Autodesk Inventor part; units mm, degrees
(part 2 of 2)
  line L844 (-48.1002, -67.2416) -> (-49.6002, -66.3756)
  line L845 (-49.6002, -66.3756) -> (-49.6002, -64.6435)
  line L846 (-42.6002, -64.6435) -> (-42.6002, -66.3756)
  line L847 (-44.1002, -63.7775) -> (-42.6002, -64.6435)
  line L848 (-42.6002, -66.3756) -> (-44.1002, -67.2416)
  line L849 (-45.6002, -64.6435) -> (-44.1002, -63.7775)
  line L850 (-44.1002, -67.2416) -> (-45.6002, -66.3756)
  line L851 (-45.6002, -66.3756) -> (-45.6002, -64.6435)
  line L852 (-38.6002, -64.6435) -> (-38.6002, -66.3756)
  line L853 (-40.1002, -63.7775) -> (-38.6002, -64.6435)
  line L854 (-38.6002, -66.3756) -> (-40.1002, -67.2416)
  line L855 (-41.6002, -64.6435) -> (-40.1002, -63.7775)
  line L856 (-40.1002, -67.2416) -> (-41.6002, -66.3756)
  line L857 (-41.6002, -66.3756) -> (-41.6002, -64.6435)
  point P0 (0, 0)
  point P1 (-72.1002, -29.5096)
  point P2 (-70.6002, -29.5096)
  point P3 (-68.1002, -29.5096)
  point P4 (-66.6002, -29.5096)
  point P5 (-64.1002, -29.5096)
  point P6 (-62.6002, -29.5096)
  point P7 (-60.1002, -29.5096)
  point P8 (-58.6002, -29.5096)
  point P9 (-56.1002, -29.5096)
  point P10 (-54.6002, -29.5096)
  point P11 (-52.1002, -29.5096)
  point P12 (-50.6002, -29.5096)
  point P13 (-48.1002, -29.5096)
  point P14 (-46.6002, -29.5096)
  point P15 (-44.1002, -29.5096)
  point P16 (-42.6002, -29.5096)
  point P17 (-40.1002, -29.5096)
  point P18 (-38.6002, -29.5096)
  point P19 (-36.1002, -29.5096)
  point P20 (-34.6002, -29.5096)
  point P21 (-32.1002, -29.5096)
  point P22 (-30.6002, -29.5096)
  point P23 (-28.1002, -29.5096)
  point P24 (-26.6002, -29.5096)
  point P25 (-24.1002, -29.5096)
  point P26 (-22.6002, -29.5096)
  point P27 (-20.1002, -29.5096)
  point P28 (-18.6002, -29.5096)
  point P29 (-16.1002, -29.5096)
  point P30 (-14.6002, -29.5096)
  point P31 (-12.1002, -29.5096)
  point P32 (-10.6002, -29.5096)
  point P33 (-8.1002, -29.5096)
  point P34 (-6.6002, -29.5096)
  point P35 (-72.1002, -33.5096)
  point P36 (-70.6002, -33.5096)
  point P37 (-68.1002, -33.5096)
  point P38 (-66.6002, -33.5096)
  point P39 (-64.1002, -33.5096)
  point P40 (-62.6002, -33.5096)
  point P41 (-60.1002, -33.5096)
  point P42 (-58.6002, -33.5096)
  point P43 (-56.1002, -33.5096)
  point P44 (-54.6002, -33.5096)
  point P45 (-52.1002, -33.5096)
  point P46 (-50.6002, -33.5096)
  point P47 (-48.1002, -33.5096)
  point P48 (-46.6002, -33.5096)
  point P49 (-44.1002, -33.5096)
  point P50 (-42.6002, -33.5096)
  point P51 (-40.1002, -33.5096)
  point P52 (-38.6002, -33.5096)
  point P53 (-36.1002, -33.5096)
  point P54 (-34.6002, -33.5096)
  point P55 (-32.1002, -33.5096)
  point P56 (-30.6002, -33.5096)
  point P57 (-28.1002, -33.5096)
  point P58 (-26.6002, -33.5096)
  point P59 (-24.1002, -33.5096)
  point P60 (-22.6002, -33.5096)
  point P61 (-20.1002, -33.5096)
  point P62 (-18.6002, -33.5096)
  point P63 (-16.1002, -33.5096)
  point P64 (-14.6002, -33.5096)
  point P65 (-12.1002, -33.5096)
  point P66 (-10.6002, -33.5096)
  point P67 (-8.1002, -33.5096)
  point P68 (-6.6002, -33.5096)
  point P69 (-72.1002, -37.5096)
  point P70 (-70.6002, -37.5096)
  point P71 (-68.1002, -37.5096)
  point P72 (-66.6002, -37.5096)
  point P73 (-64.1002, -37.5096)
  point P74 (-62.6002, -37.5096)
  point P75 (-60.1002, -37.5096)
  point P76 (-58.6002, -37.5096)
  point P77 (-56.1002, -37.5096)
  point P78 (-54.6002, -37.5096)
  point P79 (-52.1002, -37.5096)
  point P80 (-50.6002, -37.5096)
  point P81 (-48.1002, -37.5096)
  point P82 (-46.6002, -37.5096)
  point P83 (-44.1002, -37.5096)
  point P84 (-42.6002, -37.5096)
  point P85 (-40.1002, -37.5096)
  point P86 (-38.6002, -37.5096)
  point P87 (-36.1002, -37.5096)
  point P88 (-34.6002, -37.5096)
  point P89 (-32.1002, -37.5096)
  point P90 (-30.6002, -37.5096)
  point P91 (-28.1002, -37.5096)
  point P92 (-26.6002, -37.5096)
  point P93 (-24.1002, -37.5096)
  point P94 (-22.6002, -37.5096)
  point P95 (-20.1002, -37.5096)
  point P96 (-18.6002, -37.5096)
  point P97 (-16.1002, -37.5096)
  point P98 (-14.6002, -37.5096)
  point P99 (-12.1002, -37.5096)
  point P100 (-10.6002, -37.5096)
  point P101 (-8.1002, -37.5096)
  point P102 (-6.6002, -37.5096)
  point P103 (-72.1002, -41.5096)
  point P104 (-70.6002, -41.5096)
  point P105 (-68.1002, -41.5096)
  point P106 (-66.6002, -41.5096)
  point P107 (-64.1002, -41.5096)
  point P108 (-62.6002, -41.5096)
  point P109 (-60.1002, -41.5096)
  point P110 (-58.6002, -41.5096)
  point P111 (-56.1002, -41.5096)
  point P112 (-54.6002, -41.5096)
  point P113 (-52.1002, -41.5096)
  point P114 (-50.6002, -41.5096)
  point P115 (-48.1002, -41.5096)
  point P116 (-46.6002, -41.5096)
  point P117 (-44.1002, -41.5096)
  point P118 (-42.6002, -41.5096)
  point P119 (-40.1002, -41.5096)
  point P120 (-38.6002, -41.5096)
  point P121 (-36.1002, -41.5096)
  point P122 (-34.6002, -41.5096)
  point P123 (-32.1002, -41.5096)
  point P124 (-30.6002, -41.5096)
  point P125 (-28.1002, -41.5096)
  point P126 (-26.6002, -41.5096)
  point P127 (-24.1002, -41.5096)
  point P128 (-22.6002, -41.5096)
  point P129 (-20.1002, -41.5096)
  point P130 (-18.6002, -41.5096)
  point P131 (-16.1002, -41.5096)
  point P132 (-14.6002, -41.5096)
  point P133 (-12.1002, -41.5096)
  point P134 (-10.6002, -41.5096)
  point P135 (-8.1002, -41.5096)
  point P136 (-6.6002, -41.5096)
  point P137 (-72.1002, -45.5096)
  point P138 (-70.6002, -45.5096)
  point P139 (-68.1002, -45.5096)
  point P140 (-66.6002, -45.5096)
  point P141 (-64.1002, -45.5096)
  point P142 (-62.6002, -45.5096)
  point P143 (-60.1002, -45.5096)
  point P144 (-58.6002, -45.5096)
  point P145 (-56.1002, -45.5096)
  point P146 (-54.6002, -45.5096)
  point P147 (-52.1002, -45.5096)
  point P148 (-50.6002, -45.5096)
  point P149 (-48.1002, -45.5096)
  point P150 (-46.6002, -45.5096)
  point P151 (-44.1002, -45.5096)
  point P152 (-42.6002, -45.5096)
  point P153 (-40.1002, -45.5096)
  point P154 (-38.6002, -45.5096)
  point P155 (-36.1002, -45.5096)
  point P156 (-34.6002, -45.5096)
  point P157 (-32.1002, -45.5096)
  point P158 (-30.6002, -45.5096)
  point P159 (-28.1002, -45.5096)
  point P160 (-26.6002, -45.5096)
  point P161 (-24.1002, -45.5096)
  point P162 (-22.6002, -45.5096)
  point P163 (-20.1002, -45.5096)
  point P164 (-18.6002, -45.5096)
  point P165 (-16.1002, -45.5096)
  point P166 (-14.6002, -45.5096)
  point P167 (-12.1002, -45.5096)
  point P168 (-10.6002, -45.5096)
  point P169 (-8.1002, -45.5096)
  point P170 (-6.6002, -45.5096)
  point P171 (-66.6002, -45.5096)
  point P172 (-68.1002, -45.5096)
  point P173 (-62.6002, -45.5096)
  point P174 (-64.1002, -45.5096)
  point P175 (-58.6002, -45.5096)
  point P176 (-60.1002, -45.5096)
  point P177 (-54.6002, -45.5096)
  point P178 (-56.1002, -45.5096)
  point P179 (-50.6002, -45.5096)
  point P180 (-52.1002, -45.5096)
  point P181 (-46.6002, -45.5096)
  point P182 (-48.1002, -45.5096)
  point P183 (-42.6002, -45.5096)
  point P184 (-44.1002, -45.5096)
  point P185 (-38.6002, -45.5096)
  point P186 (-40.1002, -45.5096)
  point P187 (-70.6002, -49.5096)
  point P188 (-72.1002, -49.5096)
  point P189 (-66.6002, -49.5096)
  point P190 (-68.1002, -49.5096)
  point P191 (-62.6002, -49.5096)
  point P192 (-64.1002, -49.5096)
  point P193 (-58.6002, -49.5096)
  point P194 (-60.1002, -49.5096)
  point P195 (-54.6002, -49.5096)
  point P196 (-56.1002, -49.5096)
  point P197 (-50.6002, -49.5096)
  point P198 (-52.1002, -49.5096)
  point P199 (-46.6002, -49.5096)
  dimension "d5" = 31
  dimension "d6" = 24
  dimension "d7" = 7
  dimension "d8" = 4
  dimension "d9" = 7.5
  dimension "d10" = 5
  dimension "d11" = 4
  dimension "d12" = 9
  dimension "d13" = 4
  dimension "d14" = 4
  dimension "d15" = 3
  dimension "d16" = 3
  dimension "d31" = 5
  dimension "d32" = 3
  dimension "d33" = 5
  dimension "d36" = 4
  dimension "d39" = 4
  dimension "d44" = 4
  dimension "d47" = 4
  constraints: 1672 end point, 5 horizontal, 3 perpendicular, 2 centre point, 2 parallel, 2 vertical, 1 coincident, 1 midpoint, 1931 other
  measures "d5" distance of L1.end L2.end
  measures "d6" distance of L0.end L1.end
  measures "d7" distance between parallel lines of L15 L2
  measures "d8" distance between parallel lines of L17 L1
  measures "d9" diameter of A4
  measures "d10" diameter of A5
  measures "d11" distance from line of A4.centre L3
  measures "d12" distance from line of A4.centre L15
  measures "d13" distance between parallel lines of L0 L26
  measures "d14" distance between parallel lines of L2 L27
  measures "d15" distance between parallel lines of L3 L28
  measures "d16" distance between parallel lines of L1 L29
  measures "d31" distance from line of L11 point (-72.1, -29.51)
  measures "d32" distance between parallel lines of L35 L32
  measures "d33" distance from line of point (-72.1, -29.51) L7
  measures "d36" distance of L30.end L36.start
  measures "d39" distance of L30.end L132.start
  measures "d44" distance of L441.start L540.start
  measures "d47" distance of L441.start L588.start
extrude "Wyciągnięcie proste2" add sketch "Szkic2" along normal blind 3.5 contours L0 L1 L2 L3
chamfer "Faza1" distance 5 angle 45 2 edges at (31.6002, -53.0096, -1.75) (6.6002, -53.0096, -1.75)
fillet "Zaokrąglenie2" radius 1.5 10 edges at (34.6002, -49.0096, -1.75) (3.6002, -49.0096, -1.75) (6.6002, -58.0096, -1.75) (6.6002, -69.0096, -1.75) (3.6002, -73.0096, -1.75) (34.6002, -73.0096, -1.75) (31.6002, -69.0096, -1.75) (31.6002, -58.0096, -1.75) (26.6002, -53.0096, -1.75) (11.6002, -53.0096, -1.75)
sketch "Szkic3" plane through (0, 0, 0) normal (0, 0, -1) x (-1, 0, 0)
  arc A0 (-11.1608, -53.4489) -> (-12.2215, -53.0096) centre (-12.2215, -54.5096) ccw projected
  line L0 (-12.2215, -53.0096) -> (-25.9788, -53.0096) projected
  arc A1 (-25.9788, -53.0096) -> (-27.0395, -53.4489) centre (-25.9788, -54.5096) ccw projected
  line L1 (-27.0395, -53.4489) -> (-31.1608, -57.5702) projected
  arc A2 (-31.1608, -57.5702) -> (-31.6002, -58.6309) centre (-30.1002, -58.6309) ccw projected
  line L2 (-31.6002, -58.6309) -> (-31.6002, -67.5096) projected
  arc A3 (-31.6002, -67.5096) -> (-30.1002, -69.0096) centre (-30.1002, -67.5096) ccw projected
  line L3 (-30.1002, -69.0096) -> (-8.1002, -69.0096) projected
  arc A4 (-8.1002, -69.0096) -> (-6.6002, -67.5096) centre (-8.1002, -67.5096) ccw projected
  line L4 (-6.6002, -67.5096) -> (-6.6002, -58.6309) projected
  arc A5 (-6.6002, -58.6309) -> (-7.0395, -57.5702) centre (-8.1002, -58.6309) ccw projected
  line L5 (-7.0395, -57.5702) -> (-11.1608, -53.4489) projected
  point P0 (0, 0)
extrude "Wyciągnięcie proste3" cut sketch "Szkic3" against normal blind 17
extrude "Wyciągnięcie proste4" add sketch "Szkic2" along normal blind 1 contours A4
extrude "Wyciągnięcie proste5" add sketch "Szkic2" along normal blind 5 contours A5
fillet "Zaokrąglenie3" radius 2.5 1 edges at (41.1002, -71.0096, -5)
extrude "Wyciągnięcie proste6" cut sketch "Szkic2" against normal blind 2 contours L30 L31 L32 L33 L34 L35 | L36 L38 L40 L41 L39 L37 | L42 L44 L46 L47 L45 L43 | L48 L50 L52 L53 L51 L49 | L54 L56 L58 L59 L57 L55 | L60 L62 L64 L65 L63 L61 | L66 L68 L70 L71 L69 L67 | L72 L74 L76 L77 L75 L73 | L78 L80 L82 L83 L81 L79 | L84 L86 L88 L89 L87 L85 | L90 L92 L94 L95 L93 L91 | L96 L98 L100 L101 L99 L97 | L102 L104 L106 L107 L105 L103 | L108 L110 L112 L113 L111 L109 | L114 L116 L118 L119 L117 L115 | L120 L122 L124 L125 L123 L121 | L126 L128 L130 L131 L129 L127 | L132 L134 L136 L137 L135 L133 | L138 L140 L142 L143 L141 L139 | L144 L146 L148 L149 L147 L145 | L150 L152 L154 L155 L153 L151 | L156 L158 L160 L161 L159 L157 | L162 L164 L166 L167 L165 L163 | L168 L170 L172 L173 L171 L169 | L174 L176 L178 L179 L177 L175 | L180 L182 L184 L185 L183 L181 | L186 L188 L190 L191 L189 L187 | L192 L194 L196 L197 L195 L193 | L198 L200 L202 L203 L201 L199 | L204 L206 L208 L209 L207 L205 | L210 L212 L214 L215 L213 L211 | L216 L218 L220 L221 L219 L217 | L222 L224 L226 L227 L225 L223 | L228 L230 L232 L233 L231 L229 | L234 L236 L238 L239 L237 L235 | L240 L242 L244 L245 L243 L241 | L246 L248 L250 L251 L249 L247 | L252 L254 L256 L257 L255 L253 | L258 L260 L262 L263 L261 L259 | L264 L266 L268 L269 L267 L265 | L270 L272 L274 L275 L273 L271 | L276 L278 L280 L281 L279 L277 | L282 L284 L286 L287 L285 L283 | L288 L290 L292 L293 L291 L289 | L294 L296 L298 L299 L297 L295 | L300 L302 L304 L305 L303 L301 | L306 L308 L310 L311 L309 L307 | L312 L314 L316 L317 L315 L313 | L318 L320 L322 L323 L321 L319 | L324 L326 L328 L329 L327 L325 | L330 L332 L334 L335 L333 L331 | L336 L338 L340 L341 L339 L337 | L342 L344 L346 L347 L345 L343 | L348 L350 L352 L353 L351 L349 | L354 L356 L358 L359 L357 L355 | L360 L362 L364 L365 L363 L361 | L366 L368 L370 L371 L369 L367 | L372 L374 L376 L377 L375 L373 | L378 L380 L382 L383 L381 L379 | L384 L386 L388 L389 L387 L385 | L390 L392 L394 L395 L393 L391 | L396 L398 L400 L401 L399 L397 | L402 L404 L406 L407 L405 L403 | L408 L410 L412 L413 L411 L409 | L414 L416 L418 L419 L417 L415 | L420 L422 L424 L425 L423 L421 | L426 L428 L430 L431 L429 L427 | L432 L434 L436 L437 L435 L433 | L438 L440 L442 L443 L441 L439 | L444 L446 L448 L449 L447 L445 | L450 L452 L454 L455 L453 L451 | L456 L458 L460 L461 L459 L457 | L462 L464 L466 L467 L465 L463 | L468 L470 L472 L473 L471 L469 | L474 L476 L478 L479 L477 L475 | L480 L482 L484 L485 L483 L481 | L486 L488 L490 L491 L489 L487 | L492 L494 L496 L497 L495 L493 | L498 L500 L502 L503 L501 L499 | L504 L506 L508 L509 L507 L505 | L510 L512 L514 L515 L513 L511 | L516 L518 L520 L521 L519 L517 | L522 L524 L526 L527 L525 L523 | L528 L530 L532 L533 L531 L529 | L534 L536 L538 L539 L537 L535 | L588 L590 L592 L593 L591 L589 | L594 L596 L598 L599 L597 L595 | L600 L602 L604 L605 L603 L601 | L606 L608 L610 L611 L609 L607 | L612 L614 L616 L617 L615 L613 | L618 L620 L622 L623 L621 L619 | L624 L626 L628 L629 L627 L625 | L630 L632 L634 L635 L633 L631 | L636 L638 L640 L641 L639 L637 | L642 L644 L646 L647 L645 L643 | L648 L650 L652 L653 L651 L649 | L654 L656 L658 L659 L657 L655 | L660 L662 L664 L665 L663 L661 | L666 L668 L670 L671 L669 L667 | L672 L674 L676 L677 L675 L673 | L678 L680 L682 L683 L681 L679 | L684 L686 L688 L689 L687 L685 | L690 L692 L694 L695 L693 L691 | L696 L698 L700 L701 L699 L697 | L702 L704 L706 L707 L705 L703 | L708 L710 L712 L713 L711 L709 | L714 L716 L718 L719 L717 L715 | L720 L722 L724 L725 L723 L721 | L726 L728 L730 L731 L729 L727 | L732 L734 L736 L737 L735 L733 | L738 L740 L742 L743 L741 L739 | L744 L746 L748 L749 L747 L745 | L750 L752 L754 L755 L753 L751 | L756 L758 L760 L761 L759 L757 | L762 L764 L766 L767 L765 L763 | L768 L770 L772 L773 L771 L769 | L774 L776 L778 L779 L777 L775 | L780 L782 L784 L785 L783 L781 | L786 L788 L790 L791 L789 L787 | L792 L794 L796 L797 L795 L793 | L798 L800 L802 L803 L801 L799 | L804 L806 L808 L809 L807 L805 | L810 L812 L814 L815 L813 L811 | L816 L818 L820 L821 L819 L817 | L822 L824 L826 L827 L825 L823 | L828 L830 L832 L833 L831 L829 | L834 L836 L838 L839 L837 L835 | L840 L842 L844 L845 L843 L841 | L846 L848 L850 L851 L849 L847 | L852 L854 L856 L857 L855 L853
sketch "Szkic4" plane through (1.1002, -24.5096, 1.5) normal (0, 1, 0) x (1, 0, 0)
  line L0 (0, -280) -> (74.5, -280) projected
  line L1 (-1.5, 0) -> (-1.5, -278.5) projected
  line L2 (-1.5, -278.5) -> (0, -278.5) projected
  line L3 (0, -278.5) -> (0, 0) projected
  line L4 (0, 0) -> (-1.5, 0) projected
  line L5 (-1.5, 0) -> (-1.5, -278.5) projected
  line L6 (0, -278.5) -> (0, -280) projected
  line L7 (0, -280) -> (74.5, -280) projected
  line L8 (74.5, -280) -> (74.5, -278.5) projected
  line L9 (74.5, -278.5) -> (0, -278.5) projected
  line L10 (0, -278.5) -> (-1.5, -278.5) projected
  line L11 (0, -278.5) -> (0, -280) projected
  line L12 (-1.5, -278.5) -> (0, -278.5) projected
  arc A0 (-1.5, -278.5) -> (0, -280) centre (0, -278.5) ccw projected
  line L13 (74.5, 0) -> (74.5, 1.5) projected
  line L14 (74.5, 1.5) -> (0, 1.5) projected
  line L15 (0, 1.5) -> (0, 0) projected
  line L16 (0, 0) -> (74.5, 0) projected
  line L17 (74.5, -278.5) -> (76, -278.5) projected
  line L18 (76, -278.5) -> (76, 0) projected
  line L19 (76, 0) -> (74.5, 0) projected
  line L20 (74.5, 0) -> (74.5, -278.5) projected
  point P0 (-1.1002, 1.5)
  point P1 (5.5, -242)
  point P2 (66.5, -242)
  point P3 (69, -5.5)
  point P4 (5.5, -5.5)
  dimension "d52" = 7
  dimension "d53" = 7
  dimension "d54" = 7
  dimension "d55" = 7
  dimension "d56" = 38
  dimension "d57" = 38
  dimension "d58" = 7
  dimension "d59" = 9.5
  measures "d52" distance from line of L18 point (69, -5.5)
  measures "d53" distance from line of L14 point (69, -5.5)
  measures "d54" distance from line of L14 point (5.5, -5.5)
  measures "d55" distance from line of L1 point (5.5, -5.5)
  measures "d56" distance from line of L0 point (66.5, -242)
  measures "d57" distance from line of L0 point (5.5, -242)
  measures "d58" distance from line of L5 point (5.5, -242)
  measures "d59" distance from line of L18 point (66.5, -242)
hole "Otwór1" at (6.6002, -24.5096, 243.5) at (67.6002, -24.5096, 243.5) at (70.1002, -24.5096, 7) at (6.6002, -24.5096, 7) direction (0, -1, 0) diameter 3 depth 2.5
sketch "Szkic5" plane through (0, 0, 281.5) normal (0, 0, 1) x (1, 0, 0)
  line L0 (1.1002, -26.0096) -> (75.6002, -26.0096) projected
  line L1 (1.1002, -78.5096) -> (1.1002, -26.0096) projected
  line L2 (75.6002, -78.5096) -> (1.1002, -78.5096) projected
  line L3 (75.6002, -26.0096) -> (75.6002, -78.5096) projected
  line L4 (77.1002, -26.0096) -> (75.6002, -26.0096) projected
  line L5 (75.6002, -26.0096) -> (75.6002, -78.5096) projected
  line L6 (75.6002, -78.5096) -> (77.1002, -78.5096) projected
  line L7 (77.1002, -78.5096) -> (77.1002, -26.0096) projected
  line L8 (75.6002, -80.0096) -> (75.6002, -78.5096) projected
  line L9 (75.6002, -78.5096) -> (1.1002, -78.5096) projected
  line L10 (1.1002, -78.5096) -> (1.1002, -80.0096) projected
  line L11 (1.1002, -80.0096) -> (75.6002, -80.0096) projected
  line L12 (75.6002, -24.5096) -> (1.1002, -24.5096) projected
  line L13 (-0.3998, -26.0096) -> (-0.3998, -78.5096) projected
  line L14 (60.1002, -77.0096) -> (74.6002, -77.0096)
  line L15 (74.6002, -77.0096) -> (74.6002, -27.5096)
  line L16 (74.6002, -27.5096) -> (60.1002, -27.5096)
  line L17 (60.1002, -27.5096) -> (60.1002, -77.0096)
  line L18 (73.8502, -70.2596) -> (60.8502, -70.2596)
  line L19 (60.8502, -70.2596) -> (60.8502, -34.2596)
  line L20 (60.8502, -34.2596) -> (73.8502, -34.2596)
  line L21 (73.8502, -34.2596) -> (73.8502, -70.2596)
  circle A0 centre (25.6002, -52.2596) radius 20
  circle A1 centre (25.6002, -52.2596) radius 8
  arc A2 (5.6002, -52.2596) -> (18.0119, -54.7931) centre (15.6002, -34.9391) ccw
  arc A3 (5.6341, -53.4236) -> (18.4024, -55.7513) centre (15.6002, -34.9391) ccw
  arc A4 (16.6252, -70.1327) -> (25.0252, -60.2389) centre (5.6002, -52.2596) ccw
  arc A5 (15.6002, -69.5801) -> (24.0002, -60.0979) centre (5.6002, -52.2596) ccw
  circle A6 centre (25.6002, -52.2596) radius 20
  circle A7 centre (25.6002, -52.2596) radius 8
  arc A8 (36.5913, -68.9687) -> (32.2229, -56.7472) centre (15.6002, -69.5801) ccw
  arc A9 (35.6002, -69.5801) -> (31.5884, -57.5644) centre (15.6002, -69.5801) ccw
  circle A10 centre (25.6002, -52.2596) radius 20
  circle A11 centre (25.6002, -52.2596) radius 8
  arc A12 (45.5663, -51.0956) -> (32.7979, -48.7679) centre (35.6002, -69.5801) ccw
  arc A13 (45.6002, -52.2596) -> (33.1884, -49.726) centre (35.6002, -69.5801) ccw
  circle A14 centre (25.6002, -52.2596) radius 20
  circle A15 centre (25.6002, -52.2596) radius 8
  arc A16 (34.5752, -34.3864) -> (26.1752, -44.2803) centre (45.6002, -52.2596) ccw
  arc A17 (35.6002, -34.9391) -> (27.2002, -44.4212) centre (45.6002, -52.2596) ccw
  circle A18 centre (25.6002, -52.2596) radius 20
  circle A19 centre (25.6002, -52.2596) radius 8
  arc A20 (14.6091, -35.5504) -> (18.9774, -47.7719) centre (35.6002, -34.9391) ccw
  arc A21 (15.6002, -34.9391) -> (19.6119, -46.9547) centre (35.6002, -34.9391) ccw
  circle A22 centre (25.6002, -52.2596) radius 20
  circle A23 centre (25.6002, -52.2596) radius 8
  point P0 (0, 0)
  dimension "d67" = 14.5
  dimension "d68" = 49.5
  dimension "d69" = 55.5
  dimension "d70" = 3
  dimension "d71" = 2.5
  dimension "d74" = 36
  dimension "d75" = 13
  dimension "d76" = 0.75
  dimension "d77" = 6.75
  dimension "d80" = 27.75
  dimension "d81" = 26
  dimension "d82" = 40
  dimension "d83" = 16
  dimension "d84" = 20
  dimension "d85" = 1
  constraints: 48 point on circle, 24 centre point, 16 end point, 7 coincident, 4 parallel, 2 horizontal, 2 perpendicular
  measures "d67" distance of L16.end L15.end
  measures "d68" distance of L14.end L15.end
  measures "d69" distance between parallel lines of L12 L11
  measures "d70" distance between parallel lines of L11 L14
  measures "d71" distance between parallel lines of L7 L15
  measures "d74" distance of L18.end L19.end
  measures "d75" distance of L19.end L20.end
  measures "d76" distance between parallel lines of L17 L19
  measures "d77" distance between parallel lines of L16 L20
  measures "d80" distance from line of L11 point (25.6, -52.26)
  measures "d81" distance from line of L13 point (25.6, -52.26)
  measures "d82" diameter of A0
  measures "d83" diameter of A1
  measures "d84" radius of A2
  measures "d85" radial gap between concentric circles of A2 A3
extrude "Wyciągnięcie proste7" add sketch "Szkic5" along normal blind 8 contours L17 L16 L15 L14 | L18 L19 L20 L21
extrude "Wyciągnięcie proste8" cut sketch "Szkic5" along normal blind 10 contours L18 L19 L20 L21
extrude "Wyciągnięcie proste9" cut sketch "Szkic5" against normal blind 1 contours A0 A8 A1 A13 | A12 A1 A17 A0 | A0 A4 A1 A9 | A16 A1 A21 A0 | A0 A3 A1 A5 | A20 A1 A2 A0
sketch "Szkic6" plane through (-0.3998, -78.5096, 1.5) normal (-1, 0, 0) x (0, 0, 1)
  line L0 (0, 0) -> (0, 52.5) projected
  line L1 (278.5, 0) -> (0, 0) projected
  line L2 (278.5, 52.5) -> (278.5, 0) projected
  line L3 (0, 52.5) -> (278.5, 52.5) projected
  line L4 (0, -1.5) -> (278.5, -1.5) projected
  line L5 (278.5, 9.5) -> (0, 9.5)
  line L6 (0, 0) -> (0, 52.5) projected
  line L7 (278.5, 0) -> (278.5, 52.5) projected
  line L8 (278.5, 8.5) -> (0, 8.5)
  point P0 (-1.5, 78.5096)
  dimension "d91" = 11
  dimension "d92" = 1
  constraints: 4 end point, 4 point on line, 2 perpendicular
  measures "d91" distance between parallel lines of L5 L4
  measures "d92" distance between parallel lines of L8 L5
extrude "Wyciągnięcie proste10" cut sketch "Szkic6" against normal blind 0.3 contours L0 L5 L2 L8
